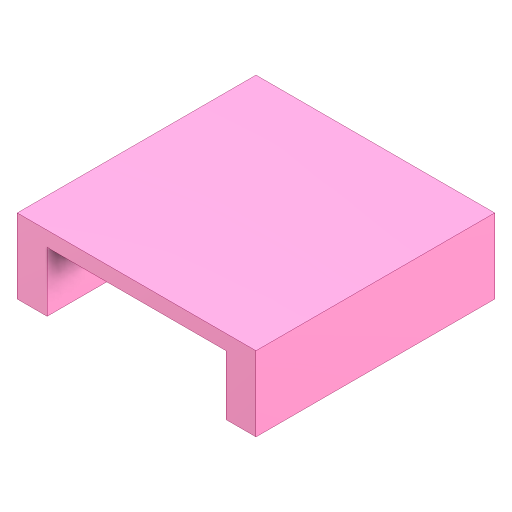
# Autodesk Inventor part: bridge_rect_final
Saved by Autodesk Inventor 2024 (Build 280153000, 153)
## iProperties
Created: 2023-08-28
Part Number: bridge_rect_final
Material: 一般
Document SubType Name: Modeling
Designer: admin
Density: 1 g/cm^3
Appearance: 平滑 - 白色
Author: admin
Autodesk Inventor part; units mm, degrees
sketch "草圖2" plane through (0, 0, 0) normal (0, 0, 1) x (1, 0, 0)
  line L0 (0, 25) -> (0, 0)
  line L1 (0, 0) -> (10, 0)
  line L2 (10, 0) -> (10, 20)
  line L3 (10, 20) -> (70, 20)
  line L4 (70, 20) -> (70, 0)
  line L5 (70, 0) -> (80, 0)
  line L6 (80, 0) -> (80, 25)
  line L7 (80, 25) -> (0, 25)
  dimension "d11" = 10
  dimension "d12" = 5
  dimension "d14" = 80
  dimension "d17" = 20
  constraints: 16 end point, 3 vertical, 2 collinear, 2 horizontal, 2 perpendicular, 1 coincident, 1 parallel
  measures "d11" distance of L0.end L1.end
  measures "d12" distance between parallel lines of L3 L7
  measures "d14" distance of L6.end L0.start
  measures "d17" distance between parallel lines of L1 L3
extrude "擠出2" add sketch "草圖2" along normal mid plane 80
ref_plane "工作平面1" through (80, 0, 40) normal (0.0872, 0, 0.9962) x (0, 1, 0)
ref_plane "工作平面2" through (80, 0, 40) normal (0.9962, 0, -0.0872) x (0, 1, 0)
ref_plane "工作平面3" through (40, 0, 40) normal (-1, 0, 0) x (0, 0, 1)
equation "\"d11\" = leg_length"
equation "\"d12\" = thickness"
equation "\"d14\" = width"
equation "\"d17\" = height"
equation "\"d15\" = length"
equation "\"width\" = 80 * ratio"
equation "\"height\" = 20 * ratio"
equation "\"length\" = width"
equation "\"leg_length\" = ratio"
equation "\"thickness\" = 5 * ratio"
equation "\"ratio\" = 1"
